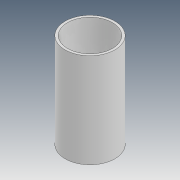
# Autodesk Inventor part: FtoF
Saved by Autodesk Inventor 2020 (Build 240168000, 168)
## iProperties
Created: 2020-05-15
Part Number: FtoF
Material: Generic
Document SubType Name: Modeling
Designer: Theo Cominotto
Density: 1 g/cm^3
Appearance: Default
Author: Theo Cominotto
Autodesk Inventor part; units mm, degrees
ref_plane "YZ Plane" through (0, 0, 0) normal (1, 0, 0) x (0, 1, 0)
ref_plane "XZ Plane" through (0, 0, 0) normal (0, 1, 0) x (-1, 0, 0)
ref_plane "XY Plane" through (0, 0, 0) normal (0, 0, 1) x (1, 0, 0)
sketch "Sketch1" plane through (0, 0, 0) normal (0, 0, 1) x (1, 0, 0)
  line L0 (0, 0) -> (0, 21) construction
  line L1 (0, 21) -> (10.66, 21) construction
  line L2 (0, 0) -> (11.185, 0) construction
  line L3 (11.185, 0) -> (10.66, 21)
  line L4 (11.185, 0) -> (12.385, 0)
  line L5 (11.185, 0) -> (12.385, 0) construction
  line L6 (12.385, 0) -> (12.385, 26)
  line L7 (10.66, 21) -> (10.66, 26)
  line L8 (10.66, 21) -> (15.66, 21) construction
  line L9 (12.385, 26) -> (10.66, 26) construction
  line L10 (12.385, 23.5) -> (10.66, 23.5) construction
  line L11 (11.185, 47) -> (10.66, 26)
  line L12 (11.185, 47) -> (12.385, 47)
  line L13 (11.185, 47) -> (12.385, 47) construction
  line L14 (12.385, 47) -> (12.385, 21)
  line L15 (10.66, 26) -> (15.66, 26) construction
  dimension "d0" = 21
  dimension "d1" = 10.66
  dimension "d2" = 11.185
  dimension "d3" = 1.2
  dimension "d4" = 0
  dimension "d5" = 5
  dimension "d6" = 90
  constraints: 32 end point, 5 symmetric about line, 4 horizontal, 3 perpendicular, 2 equal length, 2 vertical, 1 midpoint, 1 point on line
  measures "d0" distance of L0.start L0.end
  measures "d1" distance of L0.end L1.end
  measures "d2" distance of L0.start L2.end
  measures "d3" distance of L2.end L4.end
  measures "d4" distance between parallel lines of L4 L5
  measures "d5" distance of L1.end L7.end
  measures "d6" angle of L8 L7
revolve "Revolution1" add sketch "Sketch1" angle 360 about axis through (0, 0, 0) along (0, 1, 0)
body "Solid1"
